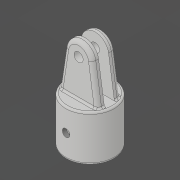
# Autodesk Inventor part: LF50-7
Saved by Autodesk Inventor 2019.4 (Build 234330000, 330)
## iProperties
Created: 2020-04-23
Part Number: LF50-7
Material: Generic
Document SubType Name: Modeling
Designer: Hannah
Density: 1 g/cm^3
Appearance: Default
Author: Hannah
Autodesk Inventor part; units mm, degrees
ref_plane "YZ Plane" through (0, 0, 0) normal (1, 0, 0) x (0, 1, 0)
ref_plane "XZ Plane" through (0, 0, 0) normal (0, 1, 0) x (-1, 0, 0)
ref_plane "XY Plane" through (0, 0, 0) normal (0, 0, 1) x (1, 0, 0)
sketch "Sketch2" plane through (0, 0, 0) normal (0, 1, 0) x (-1, 0, 0)
  circle A0 centre (0, 0) radius 22
  circle A1 centre (0, 0) radius 26.5
  dimension "d5" = 44
  dimension "d6" = 53
  constraints: 2 centre point, 2 coincident
  measures "d5" diameter of A0
  measures "d6" diameter of A1
extrude "Extrusion2" add sketch "Sketch2" along normal mid plane 50 contours A0 | A1
extrude "Extrusion3" cut sketch "Sketch2" along normal blind 20 and the other way blind 25 contours A0
hole "Hole1" at (0, 0, 0) direction (0, 0, 1) diameter 8.376 end through all thread size "M10x1.5" class "6H" standard "ISO Metric profile"
sketch "Sketch3" plane through (0, 0, 0) normal (0, 0, 1) x (1, 0, 0)
  circle A0 centre (0, 65) radius 5
  arc A1 (14.8302, 67.2503) -> (-14.8302, 67.2503) centre (0, 65) ccw
  line L0 (-21.2413, 25) -> (-14.8302, 67.2503)
  line L1 (14.8302, 67.2503) -> (21.2413, 25)
  line L2 (22, 20) -> (-22, 20) projected
  line L3 (-26.5, -25) -> (26.5, -25) projected
  line L4 (26.5, 25) -> (-26.5, 25) projected
  line L5 (-21.2413, 25) -> (21.2413, 25)
  point P0 (0, 0)
  dimension "d36" = 10
  dimension "d37" = 15
  dimension "d50" = 90
  constraints: 6 end point, 4 point on line, 2 centre point, 2 point on circle, 2 tangent, 1 coincident, 1 equal length
  measures "d36" diameter of A0
  measures "d37" radius of A1
  measures "d50" distance from line of L3 A0.centre
extrude "Extrusion5" add sketch "Sketch3" along normal mid plane 25
extrude "Extrusion6" cut sketch "Sketch3" along normal mid plane 11
fillet "Fillet2" radius 4 6 edges at (0, 80, 12.5) (18.0358, 46.1252, 12.5) (-18.0358, 46.1252, 12.5) (0, 80, -12.5) (18.0358, 46.1252, -12.5) (-18.0358, 46.1252, -12.5)
fillet "Fillet2" radius 2 2 edges at (26.5, 25, 0) (26.5, -25, 0)
fillet "Fillet3" radius 2 10 edges at (-20.0563, 25, 11.3284) (-21.2413, 25, 7) (20.0563, 25, 11.3284) (21.2413, 25, 7) (0, 25, 12.5) (20.0563, 25, -11.3284) (0, 25, -12.5) (-20.0563, 25, -11.3284) (-21.2413, 25, -7) (21.2413, 25, -7)
equation "\"d46\" = 0.5 * d7"
equation "\"d7\" = 50"
body "Solid1"
